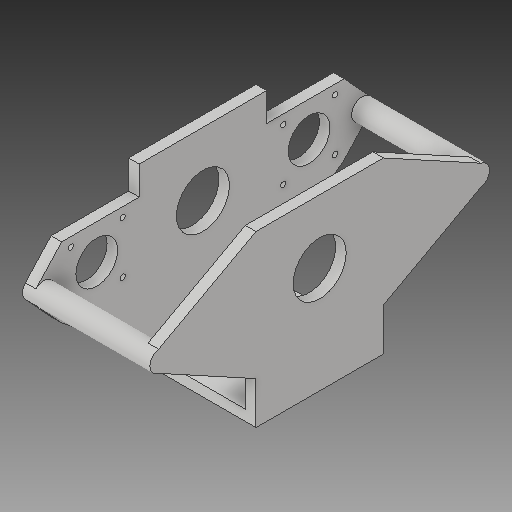
# Autodesk Inventor part: shoulder
Saved by Autodesk Inventor 2019 (Build 230136000, 136)
## iProperties
Created: 2019-02-20
Part Number: shoulder
Material: Generic
Document SubType Name: Modeling
Designer: s-2508366
Density: 1 g/cm^3
Appearance: Default
Author: s-2508366
Autodesk Inventor part; units mm, degrees
ref_plane "YZ Plane" through (0, 0, 0) normal (1, 0, 0) x (0, 1, 0)
ref_plane "XZ Plane" through (0, 0, 0) normal (0, 1, 0) x (-1, 0, 0)
ref_plane "XY Plane" through (0, 0, 0) normal (0, 0, 1) x (1, 0, 0)
sketch "Sketch1" plane through (0, 0, 0) normal (0, 1, 0) x (-1, 0, 0)
  line L0 (38.1, -38.1) -> (-38.1, -38.1)
  line L1 (-38.1, -38.1) -> (-38.1, 38.1)
  line L2 (-38.1, 38.1) -> (38.1, 38.1)
  line L3 (38.1, 38.1) -> (38.1, -38.1)
  point P0 (0, 0)
  point P1 (38.1, 0)
  point P2 (0, -38.1)
  dimension "d0" = 76.2
  dimension "d1" = 76.2
  constraints: 8 end point, 2 midpoint, 2 parallel, 1 horizontal, 1 horizontal alignment, 1 perpendicular, 1 vertical alignment
  measures "d0" distance of L0.end L1.end
  measures "d1" distance of L1.end L2.end
extrude "Extrusion1" add sketch "Sketch1" along normal blind 6.35
sketch "Sketch2" plane through (0, 6.35, 0) normal (0, 1, 0) x (1, 0, 0)
  line L0 (38.1, 38.1) -> (-38.1, 38.1) construction
  line L1 (-38.1, 38.1) -> (-38.1, -38.1) construction
  line L2 (-38.1, -38.1) -> (38.1, -38.1) construction
  line L3 (38.1, -38.1) -> (38.1, 38.1) construction
  line L4 (38.1, 38.1) -> (-38.1, 38.1) projected
  line L5 (-38.1, -38.1) -> (-31.75, -38.1)
  line L6 (-31.75, -38.1) -> (-31.75, 38.1)
  line L7 (-31.75, 38.1) -> (-38.1, 38.1)
  line L8 (-38.1, 38.1) -> (-38.1, -38.1)
  line L9 (38.1, -38.1) -> (31.75, -38.1)
  line L10 (31.75, -38.1) -> (31.75, 38.1)
  line L11 (31.75, 38.1) -> (38.1, 38.1)
  line L12 (38.1, 38.1) -> (38.1, -38.1)
  point P0 (0, 0)
  dimension "d4" = 6.35
  dimension "d5" = 6.35
  constraints: 16 end point, 4 parallel, 2 horizontal, 2 perpendicular, 2 point on line
  measures "d4" distance of L7.end L6.end
  measures "d5" distance of L10.end L11.end
extrude "Extrusion2" add sketch "Sketch2" along normal blind 95.25
sketch "Sketch5" plane through (-38.1, 0, -38.1) normal (-1, 0, 0) x (0, 0, 1)
  line L0 (76.2, 0) -> (0, 0) construction
  line L1 (76.2, 0) -> (76.2, 101.6) construction
  line L2 (0, 101.6) -> (76.2, 101.6) construction
  line L3 (0, 0) -> (0, 101.6) construction
  line L4 (-46.4, 84.5) -> (-4.4, 84.5) construction
  line L5 (-4.4, 84.5) -> (-4.4, 42.5) construction
  line L6 (-4.4, 42.5) -> (-46.4, 42.5) construction
  line L7 (-46.4, 42.5) -> (-46.4, 84.5) construction
  line L8 (-9.9, 79) -> (-40.9, 79) construction
  line L9 (-40.9, 79) -> (-40.9, 48) construction
  line L10 (-40.9, 48) -> (-9.9, 48) construction
  line L11 (-9.9, 48) -> (-9.9, 79) construction
  circle A0 centre (38.1, 63.5) radius 15.875
  line L12 (0, 6.35) -> (76.2, 6.35) construction
  line L13 (38.1, -20.32) -> (38.1, 121.92) construction
  line L14 (122.6, 84.5) -> (80.6, 84.5) construction
  line L15 (80.6, 84.5) -> (80.6, 42.5) construction
  line L16 (80.6, 42.5) -> (122.6, 42.5) construction
  line L17 (122.6, 42.5) -> (122.6, 84.5) construction
  line L18 (86.1, 79) -> (117.1, 79) construction
  line L19 (117.1, 79) -> (117.1, 48) construction
  line L20 (117.1, 48) -> (86.1, 48) construction
  line L21 (86.1, 48) -> (86.1, 79) construction
  line L22 (0, 6.35) -> (0, 101.6) projected
  line L23 (-46.4, 42.5) -> (0, 6.35)
  line L24 (-46.4, 42.5) -> (-46.4, 84.5)
  line L25 (-46.4, 84.5) -> (0, 84.5)
  point P0 (38.1, 0)
  point P1 (38.1, 0)
  point P2 (-9.9, 63.5)
  point P3 (-25.4, 63.5)
  point P4 (-25.4, 48)
  dimension "d12" = 42
  dimension "d13" = 42
  dimension "d16" = 5.5
  dimension "d17" = 31.75
  dimension "d18" = 38.1
  dimension "d19" = 63.5
  constraints: 38 end point, 12 symmetric about line, 4 coincident, 4 parallel, 4 perpendicular, 3 midpoint, 2 horizontal alignment, 2 vertical alignment, 1 centre point, 1 horizontal, 1 point on line, 3 other
  measures "d12" distance of L5.end L6.end
  measures "d13" distance of L4.end L5.end
  measures "d16" distance between parallel lines of L4 L8
  measures "d17" diameter of A0
  measures "d18" distance from line of L2 A0.centre
  measures "d19" distance of A0.centre point (-25.4, 63.5)
extrude "Extrusion3" cut sketch "Sketch5" against normal through all contours A0
extrude "Extrusion4" add sketch "Sketch5" against normal blind 6.35 contours L23 L24 L25 L22
hole "Hole1" at (-38.1, 79, -79) at (-38.1, 48, -79) at (-38.1, 48, -48) at (-38.1, 79, -48) at (-38.1, 79, 48) at (-38.1, 48, 48) at (-38.1, 48, 79) at (-38.1, 79, 79) direction (1, 0, 0) diameter 3.175 depth 25.4 tip angle 118
hole "Hole2" at (-38.1, 63.5, -63.5) direction (1, 0, 0) diameter 25 depth 25.4 tip angle 118
mirror "Mirror2" about plane through (0, 0, 0) normal (0, 0, 1) of "Hole2", "Hole1", "Extrusion4"
sketch "Sketch6" plane through (-38.1, 0, -38.1) normal (-1, 0, 0) x (0, 0, 1)
  circle A0 centre (86.1, 79) radius 1.5875 projected
  circle A1 centre (117.1, 48) radius 1.5875 projected
  circle A2 centre (117.1, 79) radius 1.5875 projected
  circle A3 centre (86.1, 48) radius 1.5875 projected
  circle A4 centre (101.6, 63.5) radius 12.5 projected
  circle A5 centre (-25.4, 63.5) radius 12.5 projected
  circle A6 centre (-9.9, 48) radius 1.5875 projected
  circle A7 centre (-40.9, 79) radius 1.5875 projected
  circle A8 centre (-40.9, 48) radius 1.5875 projected
  circle A9 centre (-9.9, 79) radius 1.5875 projected
  circle A10 centre (38.1, 63.5) radius 15.875 projected
  line L0 (76.2, 0) -> (0, 0) projected
  line L1 (76.2, 0) -> (76.2, 6.35) projected
  line L2 (122.6, 42.5) -> (76.2, 6.35) projected
  line L3 (122.6, 84.5) -> (122.6, 42.5) projected
  line L4 (76.2, 84.5) -> (122.6, 84.5) projected
  line L5 (76.2, 84.5) -> (76.2, 101.6) projected
  line L6 (0, 101.6) -> (76.2, 101.6) projected
  line L7 (0, 84.5) -> (0, 101.6) projected
  line L8 (0, 84.5) -> (-46.4, 84.5) projected
  line L9 (-46.4, 84.5) -> (-46.4, 42.5) projected
  line L10 (-46.4, 42.5) -> (0, 6.35) projected
  line L11 (0, 0) -> (0, 6.35) projected
  circle A11 centre (133.35, 63.5) radius 6.35
  line L12 (122.6, 42.5) -> (138.015, 59.1918)
  line L13 (122.6, 84.5) -> (138.015, 67.8082)
  circle A12 centre (133.35, 63.5) radius 3.175
  point P0 (38.1, 0)
  dimension "d38" = 12.7
  dimension "d39" = 31.75
  dimension "d40" = 6.35
  constraints: 4 end point, 2 centre point, 2 point on circle, 2 tangent, 1 coincident, 1 horizontal alignment
  measures "d38" diameter of A11
  measures "d39" distance of A11.centre A4.centre
  measures "d40" diameter of A12
extrude "Extrusion5" add sketch "Sketch6" against normal blind 6.35 contours L3 L13 A11 L12 | A11
mirror "Mirror3" about plane through (0, 0, 0) normal (0, 0, 1) of "Extrusion5"
sketch "Sketch7" plane through (38.1, 0, 38.1) normal (1, 0, 0) x (0, 0, -1)
  circle A0 centre (-57.15, 63.5) radius 3.175 projected
  circle A1 centre (133.35, 63.5) radius 3.175 projected
  arc A2 (-61.815, 67.8082) -> (-61.815, 59.1918) centre (-57.15, 63.5) ccw projected
  arc A3 (138.015, 59.1918) -> (138.015, 67.8082) centre (133.35, 63.5) ccw projected
  line L0 (0, 101.6) -> (76.2, 101.6) projected
  line L1 (-61.815, 67.8082) -> (0, 101.6)
  line L2 (-46.4, 42.5) -> (-61.815, 59.1918) projected
  line L3 (-61.815, 59.1918) -> (0, 25.4)
  line L4 (0, 6.35) -> (0, 101.6) projected
  circle A4 centre (133.35, 63.5) radius 3.175 construction
  line L5 (-57.15, 63.5) -> (133.35, 63.5) construction
  circle A5 centre (-57.15, 63.5) radius 3.175 construction
  arc A6 (-61.815, 67.8082) -> (-61.815, 59.1918) centre (-57.15, 63.5) ccw construction
  point P0 (38.1, 0)
  constraints: 6 end point, 2 centre point, 2 coincident, 2 point on circle, 1 horizontal, 1 point on line, 1 other
extrude "Extrusion6" add sketch "Sketch7" against normal blind 6.35 contours L1 L4 L3 A2
mirror "Mirror4" about plane through (0, 0, 0) normal (0, 0, 1) of "Extrusion6"
sketch "Sketch9" plane through (38.1, 0, 38.1) normal (1, 0, 0) x (0, 0, -1)
  circle A0 centre (133.35, 63.5) radius 3.175 projected
  circle A1 centre (-57.15, 63.5) radius 3.175 projected
  circle A2 centre (38.1, 63.5) radius 15.875 projected
  line L0 (76.2, 0) -> (0, 0) projected
  line L1 (76.2, 0) -> (76.2, 25.4) projected
  line L2 (138.015, 59.1918) -> (76.2, 25.4) projected
  arc A3 (138.015, 59.1918) -> (138.015, 67.8082) centre (133.35, 63.5) ccw projected
  line L3 (76.2, 101.6) -> (138.015, 67.8082) projected
  line L4 (0, 101.6) -> (76.2, 101.6) projected
  line L5 (0, 101.6) -> (-61.815, 67.8082) projected
  arc A4 (-61.815, 67.8082) -> (-61.815, 59.1918) centre (-57.15, 63.5) ccw projected
  line L6 (-61.815, 59.1918) -> (0, 25.4) projected
  line L7 (0, 0) -> (0, 25.4) projected
  circle A5 centre (-57.15, 63.5) radius 3.175
  circle A6 centre (133.35, 63.5) radius 3.175 projected
  circle A7 centre (133.35, 63.5) radius 3.175
  point P0 (38.1, 0)
  constraints: 2 centre point, 2 coincident, 1 concentric
extrude "Extrusion7" add sketch "Sketch9" against normal blind 6.35 contours A0 | A1
sketch "Sketch11" plane through (-38.1, 0, -38.1) normal (-1, 0, 0) x (0, 0, 1)
  circle A0 centre (-57.15, 63.5) radius 3.175 projected
  circle A1 centre (-57.15, 63.5) radius 6.35
  circle A2 centre (133.35, 63.5) radius 3.175 projected
  circle A3 centre (133.35, 63.5) radius 6.35
  arc A4 (138.015, 59.1918) -> (138.015, 67.8082) centre (133.35, 63.5) ccw projected
  arc A5 (-61.815, 67.8082) -> (-61.815, 59.1918) centre (-57.15, 63.5) ccw projected
  point P0 (38.1, 0)
  constraints: 2 centre point, 2 coincident, 2 concentric
extrude "Extrusion8" add sketch "Sketch11" against normal blind 76.2 contours A0 | A1 | A2 | A3
equation "\"d0\" = shoulder_length"
equation "\"d1\" = shoulder_width"
equation "\"d2\" = wall_thickness"
equation "\"d4\" = wall_thickness"
equation "\"d5\" = wall_thickness"
equation "\"d6\" = shoulder_height - wall_thickness"
equation "\"d18\" = bearing_distance_from_top"
equation "\"d19\" = center_distance_central_shaft"
equation "\"d22\" = wall_thickness"
equation "\"d41\" = wall_thickness"
equation "\"d43\" = wall_thickness"
equation "\"d47\" = wall_thickness"
equation "\"d49\" = shoulder_width"
equation "\"shoulder_length\" = 76.2"
equation "\"shoulder_width\" = 76.2"
equation "\"wall_thickness\" = 6.35"
equation "\"shoulder_height\" = 101.6"
equation "\"center_distance_central_shaft\" = 63.5"
equation "\"bearing_distance_from_top\" = 38.1"
body "Solid1"
